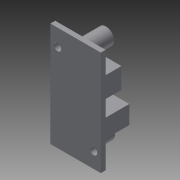
# Autodesk Inventor part: step up
Saved by Autodesk Inventor 2015 (Build 190159000, 159)
## iProperties
Created: 2015-05-05
Part Number: step up
Material: Ogólny
Document SubType Name: Modeling
Designer: Kuba
Density: 1 g/cm^3
Appearance: Domyślna
Author: Kuba
Autodesk Inventor part; units mm, degrees
ref_plane "YZ Plane" through (0, 0, 0) normal (1, 0, 0) x (0, 1, 0)
ref_plane "XZ Plane" through (0, 0, 0) normal (0, 1, 0) x (-1, 0, 0)
ref_plane "XY Plane" through (0, 0, 0) normal (0, 0, 1) x (1, 0, 0)
sketch "Szkic1" plane through (0, 0, 0) normal (0, 1, 0) x (-1, 0, 0)
  line L0 (-10.5, -21.75) -> (10.5, -21.75)
  line L1 (10.5, -21.75) -> (10.5, 21.75)
  line L2 (10.5, 21.75) -> (-10.5, 21.75)
  line L3 (-10.5, 21.75) -> (-10.5, -21.75)
  line L4 (-10.5, -21.75) -> (10.5, 21.75) construction
  line L5 (10.5, -21.75) -> (-10.5, 21.75) construction
  point P0 (0, 0)
  dimension "d0" = 21
  dimension "d1" = 43.5
  constraints: 12 end point, 2 midpoint, 2 parallel, 1 horizontal, 1 perpendicular
  measures "d0" distance of L2.end L1.end
  measures "d1" distance of L1.end L0.end
extrude "Wyciągnięcie proste1" add sketch "Szkic1" along normal blind 2
sketch "Szkic2" plane through (0, 2, 0) normal (0, 1, 0) x (1, 0, 0)
  line L0 (10.5, 21.75) -> (-10.5, 21.75) projected
  line L1 (-10.5, 21.75) -> (-10.5, -21.75) projected
  line L2 (-10.5, -21.75) -> (10.5, -21.75) projected
  line L3 (10.5, -21.75) -> (10.5, 21.75) projected
  point P0 (0, 0)
  point P1 (-7.5, -14.75)
  point P2 (7.5, 15.25)
  dimension "d4" = 3
  dimension "d5" = 7
  dimension "d6" = 6.5
  dimension "d7" = 3
  measures "d4" distance from line of L1 point (-7.5, -14.75)
  measures "d5" distance from line of L2 point (-7.5, -14.75)
  measures "d6" distance from line of L0 point (7.5, 15.25)
  measures "d7" distance from line of L3 point (7.5, 15.25)
hole "Otwór1" at (-7.5, 2, 14.75) at (7.5, 2, -15.25) direction (0, -1, 0) diameter 3 end through all
sketch "Szkic3" plane through (0, 2, 0) normal (0, 1, 0) x (1, 0, 0)
  line L0 (-7.1772, -9.2041) -> (7.109, -9.2041)
  line L1 (7.109, -9.2041) -> (7.109, -0.6113)
  line L2 (-7.1772, -9.2041) -> (-7.1772, -0.6113)
  line L3 (-7.1772, -0.6113) -> (7.109, -0.6113)
  line L4 (10.3774, 10.4592) -> (3.208, 10.4592)
  line L5 (3.208, 10.4592) -> (3.208, 2.868)
  line L6 (3.208, 2.868) -> (10.3774, 2.868)
  line L7 (10.3774, 2.868) -> (10.3774, 10.4592)
  line L8 (10.3774, 10.4592) -> (3.208, 2.868) construction
  line L9 (3.208, 10.4592) -> (10.3774, 2.868) construction
  line L10 (-5.7011, 15.0455) -> (-8.6533, 15.0455)
  line L11 (-8.6533, 15.0455) -> (-8.6533, 4.924)
  line L12 (-8.6533, 4.924) -> (-5.7011, 4.924)
  line L13 (-5.7011, 4.924) -> (-5.7011, 15.0455)
  line L14 (-5.7011, 15.0455) -> (-8.6533, 4.924) construction
  line L15 (-8.6533, 15.0455) -> (-5.7011, 4.924) construction
  circle A0 centre (0.6572, -16.8759) radius 3.3835
  circle A1 centre (1.2574, 17.1015) radius 3.1458
  point P0 (0, 0)
  point P1 (6.7927, 6.6636)
  point P2 (-7.1772, 9.9848)
  constraints: 32 end point, 4 midpoint, 4 parallel, 4 perpendicular, 3 horizontal, 2 centre point, 1 vertical
extrude "Wyciągnięcie proste2" add sketch "Szkic3" along normal blind 10
